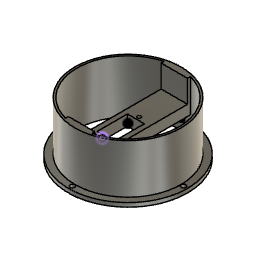
BASE v6 (Autodesk Fusion 360 design; units mm, degrees)
Autodesk Fusion 360 part; units mm, degrees
sketch "스케치1" plane through (0, 0, 0) normal (0, 0, 1) x (1, 0, 0)
  circle A0 centre (0, 0) radius 45
  dimension "d1" = 90
  constraint coincident A0.centre origin
  measures "d1" diameter of A0
extrude "돌출1" add sketch "스케치1" along normal blind 3 makes body 1
sketch "스케치2" plane through (0, 0, 3) normal (0, 0, 1) x (-1, 0, 0)
  circle A0 centre (0, 0) radius 40
  dimension "d4" = 80
  constraint coincident A0.centre origin
  measures "d4" diameter of A0
extrude "돌출2" add sketch "스케치2" along normal blind 20 bodies 1
sketch "스케치7" plane through (0, 0, 23) normal (0, 0, 1) x (-1, 0, 0)
  circle A0 centre (0, 0) radius 38.5
  line L0 (-10, 37.1786) -> (-10, -37.1786)
  line L1 (10, -37.1786) -> (10, 37.1786)
  dimension "d12" = 77
  constraint coincident A0.centre origin
  constraint parallel L0 L1
  constraint coincident A0 L0.start
  constraint coincident A0 L1.end
  constraint coincident A0 L0.end
  constraint coincident A0 L1.start
  measures "d12" diameter of A0
extrude "돌출5" cut sketch "스케치7" against normal blind 30 contours A0 L1 | A0 L0 bodies 1
sketch "스케치8" plane through (0, 0, 0) normal (0, 0, -1) x (1, 0, 0)
  line L0 (10, -37.1786) -> (10, 37.1786)
  line L1 (-10, 37.1786) -> (-10, -37.1786)
  arc A0 (-10, -37.1786) -> (10, -37.1786) centre (0, 0) ccw
  arc A1 (10, 37.1786) -> (-10, 37.1786) centre (0, 0) ccw
  dimension "d15" = 77
  constraint parallel L0 L1
  constraint coincident A0.centre A1.centre
  constraint coincident L0.end A0
  constraint concentric A0 A1
  measures "d15" diameter of A0
extrude "돌출6" cut sketch "스케치8" against normal blind 15 bodies 1
sketch "스케치9" plane through (0, 0, 23) normal (0, 0, 1) x (-1, 0, 0)
  circle A0 centre (0, 0) radius 0.8325
  constraint coincident A0.centre origin
sketch "스케치10" plane through (0, 0, 23) normal (0, 0, 1) x (1, 0, 0)
  line L0 (6.4, 5.95) -> (-6.4, 5.95)
  line L1 (-6.4, 5.95) -> (-6.4, -16.85)
  line L2 (-6.4, -16.85) -> (6.4, -16.85)
  line L3 (6.4, -16.85) -> (6.4, 5.95)
  point P0 (0, -5.45)
  constraint horizontal L0
  constraint perpendicular L0 L1
  constraint parallel L0 L2
  constraint parallel L1 L3
extrude "돌출7" cut sketch "스케치10" against normal blind 20 bodies 1
sketch "스케치11" plane through (0, 0, 23) normal (0, 0, 1) x (-1, 0, 0)
  circle A0 centre (0, -8.45) radius 1.3
  line L0 (6.4, -5.95) -> (-6.4, -5.95)
  circle A1 centre (0, 19.35) radius 1.3
  line L1 (-6.4, 16.85) -> (6.4, 16.85)
  dimension "d23" = 2.6
  dimension "d25" = 2.6
  measures "d23" diameter of A0
  measures "d25" diameter of A1
extrude "돌출8" cut sketch "스케치11" against normal blind 20 bodies 1
sketch "스케치12" plane through (0, 0, 23) normal (0, 0, 1) x (-1, 0, 0)
  circle A0 centre (0, 0) radius 40
  circle A1 centre (0, 0) radius 38.5
  dimension "d29" = 80
  dimension "d30" = 77
  constraint coincident A0.centre A1.centre
  constraint concentric A0 A1
  measures "d29" diameter of A0
  measures "d30" diameter of A1
surface "돌출9" add extruded along (0, 0, 1) between 0 and 18 profiles "스케치12" section 1 separate body makes body 2 at (-39.9503, 1.9938, 35)
sketch "스케치13" plane through (0, 0, 0) normal (0, 1, 0) x (1, 0, 0)
  circle A0 centre (0, -10) radius 5
  dimension "d33" = 10
  measures "d33" diameter of A0
extrude "돌출10" cut sketch "스케치13" along normal blind 50 bodies 1
sketch "스케치14" plane through (0, 0, 0) normal (0, 0, -1) x (1, 0, 0)
  circle A0 centre (0, -42) radius 1.75
  dimension "d36" = 3.5
  measures "d36" diameter of A0
extrude "돌출11" cut sketch "스케치14" against normal blind 10 bodies 1
sketch "스케치15" plane through (0, 0, 0) normal (0, 0, 1) x (1, 0, 0)
sketch "스케치16" plane through (0, 0, 0) normal (0, 0, -1) x (1, 0, 0)
  circle A0 centre (-42, 0) radius 1.75
  dimension "d41" = 3.5
  measures "d41" diameter of A0
extrude "돌출12" cut sketch "스케치16" against normal blind 10 bodies 1
sketch "스케치17" plane through (0, 0, 0) normal (0, 0, -1) x (1, 0, 0)
  circle A0 centre (0, 42) radius 1.75
  dimension "d44" = 3.5
  measures "d44" diameter of A0
extrude "돌출13" cut sketch "스케치17" against normal blind 10 bodies 1
sketch "스케치18" plane through (0, 0, 0) normal (0, 0, 1) x (1, 0, 0)
  circle A0 centre (42, 0) radius 1.75
  dimension "d47" = 3.5
  measures "d47" diameter of A0
extrude "돌출14" cut sketch "스케치18" along normal blind 10 bodies 1
delete_face "SurfaceDeleteFace1" leaving the opening 1 faces at (38.4521, -1.9191, 35) on bodies 2
delete_face "SurfaceDeleteFace2" leaving the opening 1 faces at (39.8012, -3.9827, 35) on bodies 2
sketch "스케치19" plane through (0, 0, 23) normal (0, 0, 1) x (-1, 0, 0)
  circle A0 centre (0, 19.35) radius 1.3
extrude "돌출15" add 1 faces at (-4.3481, 28.9385, 23) along direction (0, 0, 1) blind 17 on bodies 1 bodies 1
sketch "스케치20" plane through (0, 0, 40) normal (0, 0, 1) x (-1, 0, 0)
  line L0 (-10, 35) -> (10, 35)
  line L1 (10, 35) -> (10, -35)
  line L2 (10, -35) -> (-10, -35)
  line L3 (-10, -35) -> (-10, 35)
  constraint horizontal L0
  constraint vertical L1
  constraint horizontal L2
  constraint vertical L3
extrude "돌출16" cut sketch "스케치20" against normal blind 17 bodies 1
sketch "스케치21" plane through (0, 0, 40) normal (0, 0, 1) x (-1, 0, 0)
sketch "스케치22" plane through (0, 0, 0) normal (0, 1, 0) x (1, 0, 0)
sketch "스케치23" plane through (0, 0, 0) normal (0, 0, 1) x (1, 0, 0)
sketch "스케치3" plane through (0, 0, 23) normal (0, 0, 1) x (-1, 0, 0)
  line L0 (10, 37.1786) -> (10, -37.1786)
  line L1 (-10, -37.1786) -> (-10, 37.1786)
  arc A0 (-10, 37.1786) -> (-10, -37.1786) centre (0, 0) ccw
  arc A1 (10, -37.1786) -> (10, 37.1786) centre (0, 0) ccw
  constraint coincident A0.centre A1.centre
  constraint vertical L0
  constraint vertical L1
  constraint concentric A0 A1
extrude "돌출3" [suppressed]
sketch "스케치4" plane through (10, 0, 0) normal (1, 0, 0) x (0, 1, 0)
sketch "스케치5" plane through (0, 0, 0) normal (0, 0, -1) x (1, 0, 0)
  line L0 (10, -37.1786) -> (10, 37.1786)
  line L1 (-10, 37.1786) -> (-10, -37.1786)
  arc A0 (10, 37.1786) -> (-10, 37.1786) centre (0, 0) ccw
  arc A1 (-10, -37.1786) -> (10, -37.1786) centre (0, 0) ccw
  dimension "d9" = 77
  constraint coincident A0.centre A1.centre
  constraint parallel L0 L1
  constraint concentric A0 A1
  measures "d9" diameter of A0
extrude "돌출4" [suppressed]
sketch "스케치6" plane through (10, 0, 0) normal (1, 0, 0) x (0, 1, 0)
  line L0 (38.5, 20) -> (37.1786, 20)
  line L1 (37.1786, 20) -> (-37.1786, 20)
  line L2 (-37.1786, 20) -> (-38.5, 20)
  line L3 (-37.1786, 20) -> (37.1786, 20)
